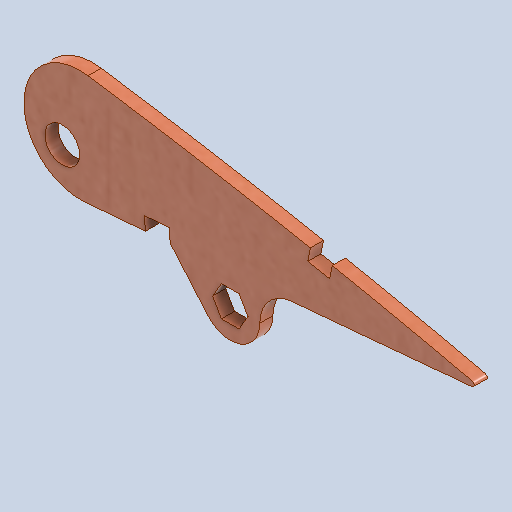
# Autodesk Inventor part: 2P.03.01.07.JW.FlapRibMid
Saved by Autodesk Inventor 2025.2 (Build 292293000, 293)
## iProperties
Created: 2024-12-05
Part Number: 2P.03.01.07.JW.FlapRibMid
Material: Wood (Walnut)
Document SubType Name: Modeling
Designer: jjrwe
Density: 0.55 g/cm^3
Appearance: Walnut - Natural Polished
Author: jjrwe
Autodesk Inventor part; units mm, degrees
ref_plane "YZ Plane" through (0, 0, 0) normal (1, 0, 0) x (0, 1, 0)
ref_plane "XZ Plane" through (0, 0, 0) normal (0, 1, 0) x (-1, 0, 0)
ref_plane "XY Plane" through (0, 0, 0) normal (0, 0, 1) x (1, 0, 0)
sketch "Sketch1" plane through (0, 0, 0) normal (0, 0, 1) x (1, 0, 0)
  spline S0 degree 2 poles (-26.5248, 6.4808) (-26.4161, 6.4647) (-26.3074, 6.4486) knots 0 0 0 1 1 1
  line L0 (-26.3296, 6.4519) -> (-26.2853, 6.4453) construction
  arc A0 (-26.2897, 6.4459) -> (-26.3252, 6.4512) centre (-41.887, -98.3753) ccw construction
  line L1 (-25.2117, -6.7841) -> (-24.9641, -9.7739)
  line L2 (-24.9641, -9.7739) -> (-19.2983, -9.3048)
  line L3 (-19.2983, -9.3048) -> (-19.5458, -6.315)
  line L4 (12.2044, 2.8479) -> (12.7843, 5.7913)
  line L5 (17.2044, 1.8628) -> (12.2044, 2.8479)
  line L6 (17.7843, 4.8062) -> (17.2044, 1.8628)
  line L7 (12.7843, 5.7913) -> (17.7843, 4.8062)
  spline S1 degree 4 poles (-38.0951, 14.4901) (-32.9548, 13.7199) (-24.3789, 12.4143) (-13.058, 10.5436) (0.6417, 8.1052) (11.6287, 6.041) (21.387, 4.092) (29.8346, 2.3727) (36.815, 0.808) (43.6252, -0.5644) (47.6422, -1.771) (50.1605, -1.8369) (50.4649, -2.6789) knots 0 0 0 0 0 0.183688 0.302378 0.416104 0.523956 0.624947 0.717922 0.80148 0.87369 1 1 1 1 1
  line L8 (-19.5458, -6.315) -> (-25.2117, -6.7841)
  arc A1 (-38.0951, 14.4901) -> (-38.9531, -10.9139) centre (-39.9909, 1.8376) ccw
  line L9 (-39.9909, 1.8376) -> (-39.9909, -2.1624)
  line L10 (-39.9909, -2.1624) -> (-43.9909, -2.1624)
  circle A2 centre (-43.9909, -2.1624) radius 4
  arc A3 (-10.6702, -19.3385) -> (1.1997, -14.9369) centre (-5.5514, -14.9369) ccw
  circle A4 centre (-5.5514, -14.9369) radius 3.5
  line L11 (-19.2983, -9.3048) -> (-10.6702, -19.3385)
  arc A5 (8.586, -6.9273) -> (1.1997, -14.9369) centre (9.2356, -14.9369) ccw
  spline S2 degree 4 poles (-38.9531, -10.9139) (-33.23, -10.4482) (-24.9952, -9.78) (-22.9103, -9.6058) (-19.2983, -9.3048) knots 0 0 0 0 0 1 1 1 1 1
  spline S3 degree 4 poles (8.4911, -6.9355) (10.4946, -6.7611) (14.9368, -6.3715) (21.4309, -5.7906) (29.3954, -5.096) (36.4972, -4.392) (43.4136, -3.8797) (47.5475, -3.2083) (50.0497, -3.468) (50.4649, -2.6789) knots 0.442408 0.442408 0.442408 0.442408 0.442408 0.523404 0.624432 0.717481 0.801136 0.873452 1 1 1 1 1
  line L12 (-21.2865, -9.4705) -> (-17.3101, -9.139) construction
  arc A6 (-17.7077, -9.1723) -> (-20.8888, -9.4375) centre (811.3613, -9974.7453) ccw construction
  line L13 (3.8187, -7.3423) -> (13.1635, -6.5288) construction
  arc A7 (4.7531, -7.2593) -> (12.2289, -6.6085) centre (-354.4003, 4161.6553) ccw construction
  line L14 (-1.5099, -14.9369) -> (-3.5307, -18.4369)
  line L15 (-3.5307, -18.4369) -> (-7.5721, -18.4369)
  line L16 (-7.5721, -18.4369) -> (-9.5928, -14.9369)
  line L17 (-9.5928, -14.9369) -> (-7.5721, -11.4369)
  line L18 (-7.5721, -11.4369) -> (-3.5307, -11.4369)
  line L19 (-3.5307, -11.4369) -> (-1.5099, -14.9369)
  point P0 (0, 0)
  point P1 (-3.4702, -1.6741)
  point P2 (-11.7791, -8.6729)
  point P3 (0.4579, -7.6289)
  point P4 (30.1549, -5.0069)
  point P5 (37.3429, -4.3499)
  point P6 (43.0189, -3.8219)
  point P7 (47.1229, -3.4349)
  point P8 (49.6039, -3.1979)
  point P9 (-24.1061, 12.3331)
  point P10 (-10.9541, 10.1431)
  point P11 (1.2109, 7.9771)
  point P12 (12.2659, 5.8921)
  point P13 (22.0909, 3.9421)
  point P14 (30.5809, 2.1811)
  point P15 (37.6519, 0.6571)
  point P16 (43.2259, -0.5789)
  point P17 (47.2519, -1.4909)
  point P18 (49.6819, -2.0489)
  point P19 (-52.7771, 2.2732)
  point P20 (8.5548, -0.5944)
  point P21 (7.5624, -0.6892)
  point P22 (5.9208, -0.844)
  point P23 (3.6504, -1.0552)
  point P24 (0.7752, -1.318)
  point P25 (-2.6688, -1.6288)
  point P26 (-6.6432, -1.9804)
  point P27 (-11.1036, -2.3668)
  point P28 (-15.9984, -2.7844)
  point P29 (-21.2724, -3.2248)
  point P30 (8.586, -0.1348)
  point P31 (7.614, 0.0884)
  point P32 (6.0036, 0.4532)
  point P33 (3.774, 0.9476)
  point P34 (0.9456, 1.5572)
  point P35 (-2.4504, 2.2616)
  point P36 (-6.3804, 3.0416)
  point P37 (-10.8024, 3.8756)
  point P38 (-15.6684, 4.742)
  point P39 (-20.9292, 5.618)
  point P40 (8.8992, -0.3868)
  point P41 (-26.868, -3.6808)
  point P42 (49.6819, -2.6199)
  point P43 (47.2519, -2.4568)
  point P44 (43.2259, -2.1907)
  point P45 (37.6519, -1.832)
  point P46 (30.5809, -1.3934)
  point P47 (22.0909, -0.8963)
  point P48 (12.2659, -0.3564)
  point P49 (1.2109, 0.2067)
  point P50 (-10.9541, 0.7703)
  point P51 (-24.1061, 1.3154)
  point P52 (-38.0951, 1.823)
  point P53 (50.4649, -3.1199)
  point P54 (-53.5871, -12.0749)
  point P55 (-52.7771, 16.5571)
  point P56 (50.4649, -2.2379)
  point P57 (8.4911, -6.9355)
  dimension "d0" = 3
  dimension "d1" = 5
  dimension "d2" = 52.7751
  dimension "d3" = 3
  dimension "d4" = 5.6658
  dimension "d5" = 4
  dimension "d6" = 4
  dimension "d7" = 8
  dimension "d8" = 7
  constraints: 40 end point, 11 point on circle, 8 centre point, 6 midpoint, 4 parallel, 3 coincident, 3 perpendicular, 2 tangent, 1 point on line, 1 vertical, 50 other
  measures "d0" distance of L6.start L6.end
  measures "d1" horizontal distance of L6.start L7.start
  measures "d2" horizontal distance of L9.start L7.start
  measures "d3" distance of L8.start L11.start
  measures "d4" horizontal distance of L8.start L1.start
  measures "d5" distance of L9.start L9.end
  measures "d6" distance of L9.end L10.end
  measures "d7" diameter of A2
  measures "d8" diameter of A4
extrude "Extrusion2" add sketch "Sketch1" along normal blind 3 contours L1 S2 A1 S1 L4 L5 L6 S3 A5 A3 L11 L3 L8
body "Solid2"
